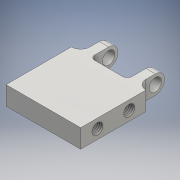
# Autodesk Inventor part: Profile_Middle_06
Saved by Autodesk Inventor 2016 (Build 200138000, 138)
## iProperties
Created: 2016-02-17
Part Number: Profile_Middle_06
Material: Aluminum 6061 T6 80 Hot Formed
Document SubType Name: Modeling
Designer: nils
Density: 2.7 g/cm^3
Appearance: Satin
Mass: 297.728 g
Surface Area: 242.248 cm^2
Volume: 110.269 cm^3
Author: nils
Autodesk Inventor part; units mm, degrees
ref_plane "YZ Plane" through (0, 0, 0) normal (1, 0, 0) x (0, 1, 0)
ref_plane "XZ Plane" through (0, 0, 0) normal (0, 1, 0) x (-1, 0, 0)
sketch "Sketch1" plane through (0, 0, 0) normal (0, 1, 0) x (-1, 0, 0)
  line L0 (0, 0) -> (80, 0)
  line L1 (80, 0) -> (80, -20)
  line L2 (80, -20) -> (0, -20)
  line L3 (0, -20) -> (0, 0)
  dimension "d0" = 80
  dimension "d1" = 20
  constraints: 8 end point, 2 parallel, 1 horizontal, 1 perpendicular
  measures "d0" distance of L1.end L2.end
  measures "d1" distance of L0.end L1.end
extrude "Extrusion1" add sketch "Sketch1" along normal blind 70
sketch "Sketch2" plane through (0, 70, 0) normal (0, 1, 0) x (1, 0, 0)
  line L0 (0, 20) -> (-80, 20) projected
  line L1 (-70, 0) -> (-60, 0)
  line L2 (-60, 0) -> (-60, 20)
  line L3 (-60, 20) -> (-70, 20)
  line L4 (-70, 20) -> (-70, 0)
  line L5 (-80, 0) -> (0, 0) projected
  line L6 (-10, 0) -> (-20, 0)
  line L7 (-20, 0) -> (-20, 20)
  line L8 (-20, 20) -> (-10, 20)
  line L9 (-10, 20) -> (-10, 0)
  line L10 (-40, 0) -> (-40, 20)
  dimension "d4" = 10
  dimension "d5" = 10
  dimension "d6" = 40
  constraints: 18 end point, 4 parallel, 3 point on line, 2 horizontal, 2 midpoint, 2 perpendicular, 1 other
  measures "d4" distance between parallel lines of L2 L4
  measures "d5" distance between parallel lines of L9 L7
  measures "d6" distance between parallel lines of L2 L7
extrude "Extrusion2" add sketch "Sketch2" along normal blind 30 contours L9 L5 L7 L0 | L2 L1 L4 L0
hole "Hole1" at (-10, 90, -10) direction (-1, 0, 0) diameter 13.5 end through all
fillet "Fillet1" radius 5 2 edges at (-20, 70, -10) (-60, 70, -10)
fillet "Fillet2" radius 10 4 edges at (-15, 100, 0) (-65, 100, 0) (-65, 100, -20) (-15, 100, -20)
sketch "Sketch3" plane through (0, 0, 0) normal (1, 0, 0) x (0, 0, -1)
  line L0 (0, 70) -> (20, 70) projected
  line L1 (10, 70) -> (10, 0)
  line L2 (0, 0) -> (20, 0) projected
  point P0 (10, 52)
  point P1 (10, 18)
  dimension "d20" = 18
  dimension "d21" = 18
  constraints: 2 end point, 2 midpoint, 2 point on line
  measures "d20" distance from line of L0 point (10, 52)
  measures "d21" distance from line of L2 point (10, 18)
hole "Hole2" at (0, 52, -10) at (0, 18, -10) direction (-1, 0, 0) diameter 11.835 depth 24 tip angle 118 thread size "M14x2" class "6H" standard "ISO Metric profile"
ref_plane "Work Plane1" through (-40, 0, 0) normal (1, 0, 0) x (0, 0, -1)
mirror "Mirror1" about plane through (-40, 0, 0) normal (1, 0, 0) of "Hole2"
fillet "Fillet3" radius 10 2 edges at (-10, 70, -10) (-70, 70, -10)
body "Solid1"
